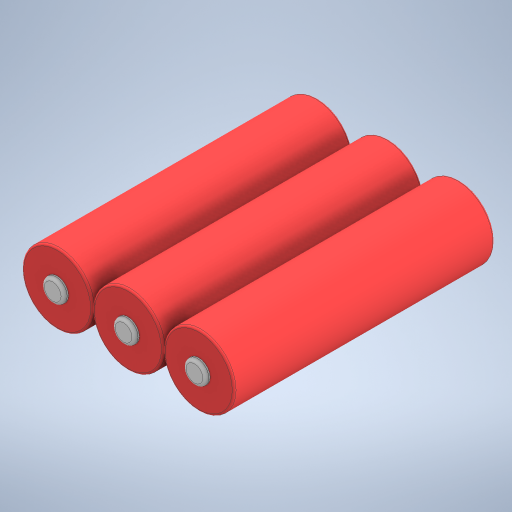
# Autodesk Inventor part: 18650배터리
Saved by Autodesk Inventor 2023.1 (Build 271208000, 208)
## iProperties
Created: 2022-08-08
Part Number: 18650배터리
Material: 일반
Document SubType Name: Modeling
Designer: fly01
Density: 1 g/cm^3
Appearance: 기본값
Author: fly01
Autodesk Inventor part; units mm, degrees
ref_plane "YZ Plane" through (0, 0, 0) normal (1, 0, 0) x (0, 1, 0)
ref_plane "XZ Plane" through (0, 0, 0) normal (0, 1, 0) x (-1, 0, 0)
ref_plane "XY Plane" through (0, 0, 0) normal (0, 0, 1) x (1, 0, 0)
sketch "스케치1" plane through (0, 0, 0) normal (0, 0, 1) x (1, 0, 0)
  circle A0 centre (0, 0) radius 9.3
  dimension "d0" = 18.6
  constraints: 1 centre point, 1 coincident
  measures "d0" diameter of A0
extrude "돌출1" add sketch "스케치1" along normal blind 68.4
fillet "모깎기1" radius 0.5 2 edges at (-9.3, 0, 68.4) (-9.3, 0, 0)
sketch "스케치4" plane through (0, 0, 68.4) normal (0, 0, 1) x (1, 0, 0)
  circle A0 centre (0, 0) radius 3
  dimension "d11" = 6
  constraints: 1 centre point, 1 coincident
  measures "d11" diameter of A0
extrude "돌출3" add sketch "스케치4" along normal blind 1.15
fillet "모깎기3" radius 0.8 1 edges at (-3, 0, 69.55)
pattern_linear "직사각형 패턴2" count 3 spacing 18.6 along (1, 0, 0) of "돌출1", "모깎기3", "돌출3", "모깎기1"
sketch "스케치5" plane through (0, 0, 68.4) normal (0, 0, 1) x (1, 0, 0)
  line L0 (0, 0) -> (7.6337, 0)
  constraints: 2 end point, 1 horizontal
